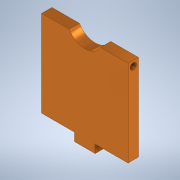
# Autodesk Inventor part: suport continuare seringa
Saved by Autodesk Inventor 2021.2 (Build 252289000, 289)
## iProperties
Created: 2024-04-19
Part Number: suport continuare seringa
Material: Gold
Document SubType Name: Modeling
Designer: cioba
Density: 19.3 g/cm^3
Appearance: Metal 1600F Hot
Author: cioba
Autodesk Inventor part; units mm, degrees
ref_plane "YZ Plane" through (0, 0, 0) normal (1, 0, 0) x (0, 1, 0)
ref_plane "XZ Plane" through (0, 0, 0) normal (0, 1, 0) x (-1, 0, 0)
ref_plane "XY Plane" through (0, 0, 0) normal (0, 0, 1) x (1, 0, 0)
sketch "Sketch1" plane through (0, 0, 0) normal (0, 0, 1) x (1, 0, 0)
  line L0 (-8.9346, 3.531) -> (-24.9346, 3.531)
  line L1 (-24.9346, 3.531) -> (-24.9346, 45.531)
  line L2 (17.0654, 45.531) -> (17.0654, 3.531)
  line L3 (17.0654, 3.531) -> (1.0654, 3.531)
  line L4 (-8.9346, -0.469) -> (1.0654, -0.469)
  line L5 (-8.9346, 3.531) -> (-8.9346, -0.469)
  line L6 (1.0654, 3.531) -> (1.0654, -0.469)
  line L7 (17.0654, 45.531) -> (3.6736, 45.531)
  line L8 (-24.9346, 45.531) -> (-11.5428, 45.531)
  arc A0 (-11.5428, 45.531) -> (3.6736, 45.531) centre (-3.9346, 49.8809) ccw
  point P0 (0, 0)
  constraints: 18 end point, 2 horizontal, 2 point on circle, 2 point on line, 1 centre point, 1 parallel, 1 perpendicular, 1 vertical
extrude "Extrusion4" add sketch "Sketch1" against normal blind 5
sketch "Sketch2" plane through (17.0654, 3.531, 0) normal (1, 0, 0) x (0, 0, -1)
  line L0 (0, 42) -> (5, 42) projected
  line L1 (0, 42) -> (0, 39.5)
  line L2 (0, 37.5859) -> (0, 42) projected
  line L3 (0, 39.5) -> (5, 39.5)
  line L4 (5, 42) -> (5, 37.5859) projected
  circle A0 centre (2.5, 39.5) radius 1.5
  point P0 (0, -3.531)
  constraints: 4 end point, 2 point on line, 1 centre point, 1 midpoint, 1 perpendicular
hole "Hole1" at (17.0654, 43.031, -2.5) direction (-1, 0, 0) diameter 3 depth 5 tip angle 118
sketch "Sketch3" plane through (-24.9346, 3.531, 0) normal (-1, 0, 0) x (0, 0, 1)
  circle A0 centre (-2.5, 39.5) radius 1.5 projected
  circle A1 centre (-2.5, 39.5) radius 1.5
  point P0 (0, -3.531)
  constraints: 1 centre point, 1 coincident
hole "Hole2" at (-24.9346, 43.031, -2.5) direction (1, 0, 0) diameter 3 depth 5 tip angle 118
body "Solid2"
